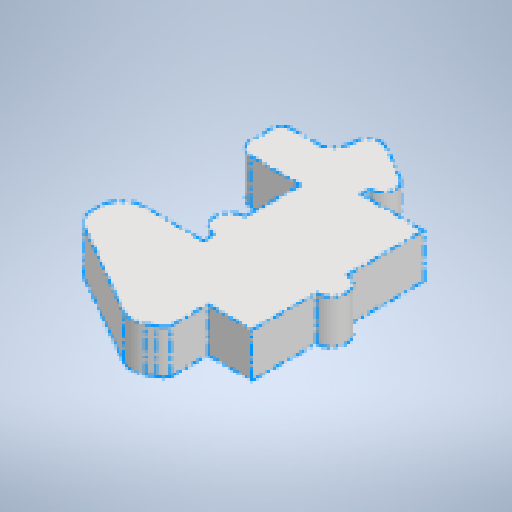
# Autodesk Inventor part: microb_connection_base
Saved by Autodesk Inventor 2024.1 (Build 281209000, 209)
## iProperties
Created: 2025-06-17
Part Number: microb_connection_base
Material: 一般
Document SubType Name: Modeling
Designer: hibik
Density: 1 g/cm^3
Appearance: 既定
Author: hibik
Autodesk Inventor part; units mm, degrees
ref_plane "YZ Plane" through (0, 0, 0) normal (1, 0, 0) x (0, 1, 0)
ref_plane "XZ Plane" through (0, 0, 0) normal (0, 1, 0) x (-1, 0, 0)
ref_plane "XY Plane" through (0, 0, 0) normal (0, 0, 1) x (1, 0, 0)
sketch "スケッチ1" plane through (0, 0, 0) normal (0, 1, 0) x (-1, 0, 0)
  line L0 (13.5, 20.5761) -> (13.5, 0) projected
  line L1 (13.5, 0) -> (40.1503, 0) projected
  arc A0 (40.1503, 0) -> (45.1503, 5) centre (40.1503, 5) ccw projected
  line L2 (45.1503, 5) -> (45.1503, 6.5367) projected
  arc A1 (45.1503, 6.5367) -> (42.6503, 10.8669) centre (40.1503, 6.5367) ccw projected
  line L3 (42.6503, 10.8669) -> (21.6525, 22.9899) projected
  arc A2 (21.6525, 22.9899) -> (16.6525, 22.9899) centre (19.1525, 18.6598) ccw projected
  line L4 (16.6525, 22.9899) -> (15.1554, 22.1256) projected
  arc A3 (15.1554, 22.1256) -> (13.5, 20.5761) centre (17.6554, 17.7954) ccw projected
  line L5 (26.5, -2.5) -> (26.5, 0) projected
  line L6 (26.5, 0) -> (13.5, 0) projected
  line L7 (13.5, 0) -> (13.5, 12) projected
  line L8 (13.5, 12) -> (3.5, 12) projected
  line L9 (3.5, 12) -> (3.5, -2.5) projected
  arc A4 (3.5, -2.5) -> (3.5, -9.5) centre (3.5, -6) ccw projected
  line L10 (3.5, -9.5) -> (3.5, -27) projected
  line L11 (3.5, -27) -> (26.5, -27) projected
  line L12 (26.5, -27) -> (26.5, -9.5) projected
  arc A5 (26.5, -9.5) -> (26.5, -2.5) centre (26.5, -6) ccw projected
  arc A6 (24.3136, -39.1968) -> (28.8136, -36.5918) centre (25.8136, -36.5988) ccw projected
  arc A7 (31.3136, -32.25) -> (28.8136, -36.5918) centre (33.8136, -36.5802) ccw projected
  line L13 (31.3136, -32.25) -> (31.7466, -32) projected
  line L14 (31.7466, -32) -> (38.871, -32) projected
  arc A8 (38.871, -32) -> (40.871, -30) centre (38.871, -30) ccw projected
  line L15 (40.871, -30) -> (40.871, -25) projected
  arc A9 (40.871, -25) -> (37.871, -22) centre (37.871, -25) ccw projected
  line L16 (37.871, -22) -> (26.5, -22) projected
  line L17 (26.5, -22) -> (26.5, -27) projected
  line L18 (26.5, -27) -> (17.8483, -27) projected
  line L19 (17.8483, -27) -> (17.8483, -29) projected
  arc A10 (17.8483, -29) -> (16.3483, -34.5981) centre (17.8483, -32) ccw projected
  line L20 (16.3483, -34.5981) -> (24.3136, -39.1968) projected
  point P0 (0, 0)
extrude "押し出し1" add sketch "スケッチ1" along normal blind 10
